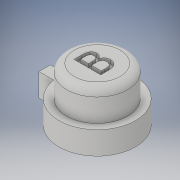
# Autodesk Inventor part: ButtonB_neu
Saved by Autodesk Inventor 2019 (Build 230136000, 136)
## iProperties
Created: 2020-09-24
Part Number: ButtonB_neu
Material: Generisch
Document SubType Name: Modeling
Designer: David
Density: 1 g/cm^3
Appearance: Vorgabe
Author: David
Autodesk Inventor part; units mm, degrees
ref_plane "YZ Plane" through (0, 0, 0) normal (1, 0, 0) x (0, 1, 0)
ref_plane "XZ Plane" through (0, 0, 0) normal (0, 1, 0) x (-1, 0, 0)
ref_plane "XY Plane" through (0, 0, 0) normal (0, 0, 1) x (1, 0, 0)
sketch "Skizze1" plane through (0, 0, 0) normal (1, 0, 0) x (0, 1, 0)
  line L0 (4, 0) -> (4, 3)
  arc A0 (4, 3) -> (3, 4) centre (3, 3) ccw
  line L1 (3, 4) -> (0, 4)
  line L2 (0, 4) -> (0, 5)
  line L3 (0, 5) -> (-3, 5)
  line L4 (-3, 5) -> (-3, 2)
  line L5 (0, 0) -> (4, 0)
  line L6 (-3, 2) -> (-3, 0)
  line L7 (-3, 0) -> (0, 0)
  point P0 (0, 2)
  dimension "d0" = 2
  dimension "d1" = 4
  dimension "d2" = 3
  dimension "d3" = 5
  dimension "d4" = 3
  dimension "d5" = 1
  dimension "d6" = 1
  constraints: 16 end point, 4 perpendicular, 2 point on circle, 2 vertical, 1 centre point, 1 horizontal, 1 point on line, 1 tangent
  measures "d0" distance of point (0, 2) L5.start
  measures "d1" distance between parallel lines of L5 L1
  measures "d2" distance of L4.end point (0, 2)
  measures "d3" distance between parallel lines of L5 L3
  measures "d4" distance of L1.start L1.end
  measures "d5" distance from line of L1.start L0
  measures "d6" horizontal distance of L1.start L0.end
revolve "Umdrehung1" add sketch "Skizze1" angle 360 about axis through (0, 0, 0) along (0, 1, 0)
sketch "Skizze2" plane through (0, 4, 0) normal (0, 1, 0) x (1, 0, 0)
  line L0 (-1.9622, -1.4344) -> (-1.9622, 1.4984) construction
  line L1 (-1.9622, 1.4984) -> (1.5378, 1.4984) construction
  line L2 (1.5378, 1.4984) -> (1.5378, -1.4344) construction
  line L3 (1.5378, -1.4344) -> (-1.9622, -1.4344) construction
  spline S0 degree 2 poles (0.4629, 1.2942) (0.7238, 1.2942) (1.1237, 1.0956) (1.2542, 0.9311) knots 0 0 0 1 2 2 2
  spline S1 degree 2 poles (1.2542, 0.9311) (1.4074, 0.7326) (1.5378, 0.2816) (1.5378, -0.0758) knots 0 0 0 1 2 2 2
  line L4 (1.5378, -0.0758) -> (1.5378, -1.0798)
  line L5 (1.5378, -1.0798) -> (-1.9622, -1.0798)
  line L6 (-1.9622, -1.0798) -> (-1.9622, -0.1523)
  spline S2 degree 2 poles (-1.9622, -0.1523) (-1.9622, 0.222) (-1.914, 0.5964) (-1.8204, 0.7666) knots 0 0 0 1 2 2 2
  spline S3 degree 2 poles (-1.8204, 0.7666) (-1.7211, 0.9566) (-1.3949, 1.1297) (-1.1737, 1.1297) knots 0 0 0 1 2 2 2
  spline S4 degree 2 poles (-1.1737, 1.1297) (-0.9269, 1.1297) (-0.5355, 0.8687) (-0.4249, 0.639) knots 0 0 0 1 2 2 2
  line L7 (-0.4249, 0.639) -> (-0.4079, 0.639)
  spline S5 degree 2 poles (-0.4079, 0.639) (-0.3228, 0.951) (0.1282, 1.2942) (0.4629, 1.2942) knots 0 0 0 1 2 2 2
  spline S6 degree 2 poles (0.4827, 0.8092) (0.2842, 0.8092) (0.0289, 0.6957) (-0.0618, 0.5255) knots 0 0 0 1 2 2 2
  spline S7 degree 2 poles (-0.0618, 0.5255) (-0.1186, 0.4149) (-0.1526, 0.154) (-0.1526, -0.0871) knots 0 0 0 1 2 2 2
  line L8 (-0.1526, -0.0871) -> (-0.1526, -0.6147)
  line L9 (-0.1526, -0.6147) -> (1.1407, -0.6147)
  line L10 (1.1407, -0.6147) -> (1.1407, -0.2374)
  spline S8 degree 2 poles (1.1407, -0.2374) (1.1407, 0.0689) (1.084, 0.4206) (0.9933, 0.5567) knots 0 0 0 1 2 2 2
  spline S9 degree 2 poles (0.9933, 0.5567) (0.8997, 0.6872) (0.6671, 0.8092) (0.4827, 0.8092) knots 0 0 0 1 2 2 2
  spline S10 degree 2 poles (-1.1084, 0.6447) (-1.2332, 0.6447) (-1.4204, 0.5596) (-1.4743, 0.466) knots 0 0 0 1 2 2 2
  spline S11 degree 2 poles (-1.4743, 0.466) (-1.5367, 0.3525) (-1.5651, 0.0774) (-1.5651, -0.1694) knots 0 0 0 1 2 2 2
  line L11 (-1.5651, -0.1694) -> (-1.5651, -0.6147)
  line L12 (-1.5651, -0.6147) -> (-0.5412, -0.6147)
  line L13 (-0.5412, -0.6147) -> (-0.5412, -0.0871)
  spline S12 degree 2 poles (-0.5412, -0.0871) (-0.5412, 0.1313) (-0.5866, 0.3383) (-0.6575, 0.449) knots 0 0 0 1 2 2 2
  spline S13 degree 2 poles (-0.6575, 0.449) (-0.7255, 0.5567) (-0.9439, 0.6447) (-1.1084, 0.6447) knots 0 0 0 1 2 2 2
  point P0 (0, 0)
  constraints: 2 other
extrude "Extrusion1" cut sketch "Skizze2" against normal blind 0.5
sketch "Skizze4" plane through (0, -3, 0) normal (0, -1, 0) x (1, 0, 0)
  line L0 (-4.889, 0.75) -> (-6.889, 0.75)
  line L1 (-6.889, 0.75) -> (-6.889, -0.75)
  line L2 (-6.889, -0.75) -> (-4.889, -0.75)
  line L3 (-4.889, -0.75) -> (-4.889, 0.75)
  point P0 (0, 0)
  dimension "d15" = 1.5
  dimension "d16" = 2
  dimension "d17" = 0.75
  constraints: 8 end point, 2 parallel, 1 horizontal, 1 perpendicular
  measures "d15" distance of L2.end L0.start
  measures "d16" distance between parallel lines of L1 L3
  measures "d17" vertical distance of L0.start point (0, 0)
extrude "Extrusion3" add sketch "Skizze4" against normal blind 3
